Autodesk Inventor part; units mm, degrees
(part 3 of 3)
  arc A13 (32.3087, 73.7581) -> (27.3087, 68.7581) centre (32.3087, 68.7581) ccw
  arc A14 (24.8087, 63.7581) -> (27.3087, 66.2581) centre (24.8087, 66.2581) ccw
  arc A15 (87.3087, 66.2581) -> (89.8087, 63.7581) centre (89.8087, 66.2581) ccw
  line L1771 (160.5067, -66.0674) -> (89.8207, -66.0674)
  line L1772 (-149.0562, -66.0674) -> (-78.3702, -66.0674)
  line L1773 (57.3207, -76.0674) -> (82.3207, -76.0674)
  line L1774 (57.3207, -76.0674) -> (32.3207, -76.0674)
  line L1775 (87.3207, -71.0674) -> (87.3207, -68.5674)
  line L1776 (27.3207, -71.0674) -> (27.3207, -68.5674)
  arc A16 (27.3207, -71.0674) -> (32.3207, -76.0674) centre (32.3207, -71.0674) ccw
  arc A17 (82.3207, -76.0674) -> (87.3207, -71.0674) centre (82.3207, -71.0674) ccw
  arc A18 (89.8207, -66.0674) -> (87.3207, -68.5674) centre (89.8207, -68.5674) ccw
  arc A19 (27.3207, -68.5674) -> (24.8207, -66.0674) centre (24.8207, -68.5674) ccw
  line L1777 (-45.8702, -76.0674) -> (-20.8702, -76.0674)
  line L1778 (-45.8702, -76.0674) -> (-70.8702, -76.0674)
  line L1779 (-15.8702, -71.0674) -> (-15.8702, -68.5674)
  line L1780 (-75.8702, -71.0674) -> (-75.8702, -68.5674)
  arc A20 (-75.8702, -71.0674) -> (-70.8702, -76.0674) centre (-70.8702, -71.0674) ccw
  arc A21 (-20.8702, -76.0674) -> (-15.8702, -71.0674) centre (-20.8702, -71.0674) ccw
  arc A22 (-13.3702, -66.0674) -> (-15.8702, -68.5674) centre (-13.3702, -68.5674) ccw
  arc A23 (-75.8702, -68.5674) -> (-78.3702, -66.0674) centre (-78.3702, -68.5674) ccw
  line L1781 (24.8207, -66.0674) -> (-13.3702, -66.0674)
  line L1782 (-13.3702, -66.0674) -> (5.7248, -66.0674)
  line L1783 (-13.3822, 63.7581) -> (5.7128, 63.7581)
  arc A24 (-149.0562, 63.7581) -> (-152.0562, 60.7286) centre (-149.0562, 60.7579) ccw
  arc A25 (163.5067, 60.7579) -> (160.4947, 63.7581) centre (160.6009, 60.8527) ccw
  arc A26 (160.5067, -66.0674) -> (163.5067, -63.0674) centre (160.5067, -63.0674) ccw
  arc A27 (-152.0562, -63.0674) -> (-149.0562, -66.0674) centre (-149.0562, -63.0674) ccw
  line L1784 (103.6297, 45.2329) -> (103.6297, 57.2329)
  line L1785 (103.6297, 57.2329) -> (108.6297, 57.2329)
  line L1786 (108.6297, 57.2329) -> (108.6297, 45.2329)
  line L1787 (108.6297, 45.2329) -> (103.6297, 45.2329)
  point P0 (0, 0)
  constraints: 3576 end point, 56 point on circle, 28 centre point, 4 point on line
extrude "Extrusion1" add sketch "Sketch1" along normal blind 2
body "Solid1"
